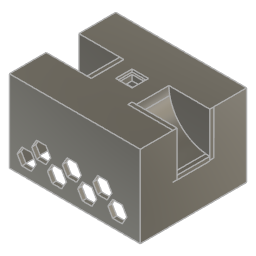
Housing_2_c v4 (Autodesk Fusion 360 archive; units mm, degrees)
design "Housing_2_c"
part number: Configuration 1
Autodesk Fusion 360 part; units mm, degrees
sketch "Sketch1" plane through (0, 0, 0) normal (0, 1, 0) x (1, 0, 0)
  line L0 (0, 0) -> (203.2, 0)
  line L1 (203.2, 0) -> (203.2, -127)
  line L2 (203.2, -127) -> (0, -127)
  line L3 (0, -127) -> (0, 0)
  dimension "d1" = 203.2
  dimension "d2" = 127
  constraint horizontal L0
  constraint vertical L1
  constraint horizontal L2
  constraint vertical L3
  constraint coincident L0.start L3.end
  measures "d1" distance of L0.start L0.end
  measures "d2" distance of L0.start L2.end
extrude "Extrude1" add sketch "Sketch1" along normal blind 165.1
sketch "Sketch3" plane through (0, 0, 0) normal (0, 0, -1) x (1, 0, 0)
  line L0 (203.2, 0) -> (0, 0)
  line L1 (0, 0) -> (0, -165.1)
  line L2 (0, -165.1) -> (203.2, -165.1)
  line L3 (203.2, -165.1) -> (203.2, 0)
  line L4 (6.35, -6.35) -> (196.85, -6.35)
  line L5 (196.85, -6.35) -> (196.85, -158.75)
  line L6 (196.85, -158.75) -> (6.35, -158.75)
  line L7 (6.35, -158.75) -> (6.35, -6.35)
  dimension "d7" = 190.5
  dimension "d8" = 152.4
  dimension "d9" = 6.35
  dimension "d10" = 6.35
  constraint horizontal L4
  constraint vertical L5
  constraint horizontal L6
  constraint vertical L7
  measures "d7" distance of L4.start L4.end
  measures "d8" distance of L4.start L6.end
  measures "d9" distance of L0 L4
  measures "d10" distance of L1 L7
extrude "Extrude2" cut sketch "Sketch3" against normal blind 114.3 contours L4 L5 L6 L7
sketch "Sketch4" plane through (0, 0, 127) normal (0, 0, 1) x (-1, 0, 0)
  line L0 (0, 0) -> (-203.2, 0)
  line L1 (-203.2, 0) -> (-203.2, -165.1)
  line L2 (-203.2, -165.1) -> (0, -165.1)
  line L3 (0, -165.1) -> (0, 0)
  line L4 (-88.9, -101.6) -> (-114.3, -101.6)
  line L5 (-114.3, -101.6) -> (-114.3, -76.2)
  line L6 (-114.3, -76.2) -> (-88.9, -76.2)
  line L7 (-88.9, -76.2) -> (-88.9, -101.6)
  line L8 (-111.125, -79.375) -> (-92.075, -79.375)
  line L9 (-92.075, -79.375) -> (-92.075, -98.425)
  line L10 (-92.075, -98.425) -> (-111.125, -98.425)
  line L11 (-111.125, -98.425) -> (-111.125, -79.375)
  line L12 (-111.125, -79.375) -> (-92.075, -98.425) construction
  line L13 (-92.075, -79.375) -> (-111.125, -98.425) construction
  point P0 (-101.6, -88.9)
  dimension "d13" = 25.4
  dimension "d14" = 25.4
  dimension "d15" = 88.9
  dimension "d16" = 76.2
  dimension "d17" = 19.05
  dimension "d18" = 19.05
  constraint horizontal L4
  constraint vertical L5
  constraint horizontal L6
  constraint vertical L7
  constraint horizontal L8
  constraint perpendicular L8 L9
  constraint parallel L8 L10
  constraint parallel L9 L11
  constraint coincident L12 P0
  constraint coincident L13 P0
  measures "d13" distance of L4.start L4.end
  measures "d14" distance of L4.start L6.end
  measures "d15" distance of L1 L5
  measures "d16" distance of L0 L6
  measures "d17" distance of L9.end L10.end
  measures "d18" distance of L8.end L9.end
extrude "Extrude3" cut sketch "Sketch4" against normal blind 4.064 contours L4 L5 L6 L7
extrude "Extrude4" cut 1 faces at (104.775, 92.075, 127) along direction (0, 0, -1) blind 12.7
ref_plane "WorkPlane1" through (101.6, 82.55, 57.15) normal (0, -1, 0) x (1, 0, 0)
sketch "Sketch5" plane through (0, 82.55, 0) normal (0, -1, 0) x (-1, 0, 0)
  circle A0 centre (-203.2569, -127.0062) radius 63.5
  circle A1 centre (-203.2569, -127.0062) radius 60.325
  dimension "d23" = 127
  dimension "d29" = 120.65
  constraint concentric A0 A1
  measures "d23" diameter of A0
  measures "d29" diameter of A1
extrude "Extrude5" cut sketch "Sketch5" along normal mid plane 50.8 contours A0 | A1
sketch "Sketch6" plane through (0, 82.55, 0) normal (0, -1, 0) x (-1, 0, 0)
  circle A0 centre (0.0225, -126.9197) radius 63.5
  dimension "d26" = 127
  measures "d26" diameter of A0
extrude "Extrude6" cut sketch "Sketch6" along normal mid plane 50.8
sketch "Sketch9" plane through (0, 82.55, 0) normal (0, -1, 0) x (-1, 0, 0)
  arc A0 (-139.7096, -126.9974) -> (-203.216, -63.5038) centre (-203.2096, -127.0038) ccw
  line L0 (-203.2096, -127.0038) -> (-139.7096, -126.9974) construction
  line L1 (-203.2096, -127.0038) -> (-203.216, -63.5038) construction
  line L2 (-203.2096, -127.0038) -> (-146.0596, -126.9981) construction
  line L3 (-203.2096, -127.0038) -> (-203.2154, -69.8538) construction
  arc A1 (-133.3596, -126.9968) -> (-203.2166, -57.1538) centre (-203.2096, -127.0038) ccw
  line L4 (-203.2096, -127.0038) -> (-133.3596, -126.9968) construction
  line L5 (-203.2096, -127.0038) -> (-203.2166, -57.1538) construction
  line L6 (-133.3596, -126.9968) -> (-139.7096, -126.9974)
  line L7 (-203.216, -63.5038) -> (-203.2166, -57.1538)
  dimension "d34" = 63.5
  dimension "d35" = 90
  dimension "d37" = 90
  dimension "d38" = 69.85
  dimension "d39" = 90
  constraint coincident L1 L3.end
  constraint coincident A0.centre L0.start
  constraint parallel L4 L6
  measures "d34" radius of A0
  measures "d35" angle of L0 L1
  measures "d37" angle of L2 L3
  measures "d38" radius of A1
  measures "d39" angle of L4 L5
extrude "Extrude8" add sketch "Sketch9" along normal mid plane 50.8
sketch "Sketch10" plane through (0, 82.55, 0) normal (0, -1, 0) x (-1, 0, 0)
  arc A0 (-0.171, -63.3672) -> (-63.4547, -127.0827) centre (0.0449, -126.8668) ccw
  line L0 (0.0449, -126.8668) -> (-0.171, -63.3672) construction
  line L1 (0.0449, -126.8668) -> (-63.4547, -127.0827) construction
  arc A1 (-0.1926, -57.0172) -> (-69.8047, -127.1043) centre (0.0449, -126.8668) ccw
  line L2 (0.0449, -126.8668) -> (-0.1926, -57.0172) construction
  line L3 (0.0449, -126.8668) -> (-69.8047, -127.1043) construction
  line L4 (-63.4547, -127.0827) -> (-69.8047, -127.1043)
  line L5 (-0.171, -63.3672) -> (-0.1926, -57.0172)
  dimension "d42" = 63.5
  dimension "d43" = 90
  dimension "d44" = 69.85
  dimension "d45" = 90
  constraint coincident A0.centre L0.start
  constraint parallel L3 L4
  measures "d42" radius of A0
  measures "d43" angle of L0 L1
  measures "d44" radius of A1
  measures "d45" angle of L2 L3
extrude "Extrude9" add sketch "Sketch10" along normal mid plane 50.8
sketch "Sketch12" plane through (0, 107.95, 0) normal (0, -1, 0) x (1, 0, 0)
  arc A0 (62.1991, 114.3) -> (63.4549, 127) centre (-0.0449, 126.8668) ccw
  line L0 (63.4549, 127) -> (0, 127)
  line L1 (0, 127) -> (0, 63.4197)
  arc A1 (0, 63.4197) -> (6.35, 63.7403) centre (-0.0225, 126.9197) ccw
  line L2 (6.35, 63.7403) -> (6.35, 114.3)
  line L3 (6.35, 114.3) -> (62.1991, 114.3)
  arc A2 (0.0585, 57.0697) -> (69.8275, 127.0007) centre (-0.0225, 126.9197) ccw
  line L4 (-0.0225, 126.9197) -> (0.0585, 57.0697) construction
  line L5 (-0.0225, 126.9197) -> (69.8275, 127.0007) construction
  line L6 (-0.0225, 126.9197) -> (69.8275, 127.0007)
  line L7 (-0.0225, 126.9197) -> (0.0585, 57.0697)
  dimension "d48" = 69.85
  dimension "d49" = 90
  constraint coincident A1.centre A2.centre
  measures "d48" radius of A2
  measures "d49" angle of L4 L5
sketch "Sketch13" plane through (0, 0, 0) normal (0, -1, 0) x (1, 0, 0)
  line L0 (203.2, 127) -> (0, 127)
  line L1 (0, 127) -> (0, 0)
  line L2 (0, 0) -> (203.2, 0)
  line L3 (203.2, 0) -> (203.2, 127)
  line L4 (34.1009, 12.754) -> (41.4333, 25.454)
  line L5 (41.4333, 25.454) -> (34.1009, 38.154)
  line L6 (34.1009, 38.154) -> (19.4362, 38.154)
  line L7 (19.4362, 38.154) -> (12.1039, 25.454)
  line L8 (12.1039, 25.454) -> (19.4362, 12.754)
  line L9 (19.4362, 12.754) -> (34.1009, 12.754)
  point P0 (26.7686, 25.454)
  dimension "d55" = 12.7
  constraint parallel L2 L9
  measures "d55" distance of P0 L9
extrude "Extrude12" cut sketch "Sketch13" against normal blind 6.35 contours L4 L5 L6 L7 L8 L9
pattern_linear "R-Pattern1" count 4 spacing 46.99 along (1, 0, 0) of "Extrude12"
sketch "Sketch14" plane through (0, 0, 0) normal (0, -1, 0) x (1, 0, 0)
  line L0 (182.4033, 25.454) -> (175.0709, 12.754)
  line L1 (175.0709, 12.754) -> (160.4062, 12.754)
  line L2 (160.4062, 12.754) -> (153.0739, 25.454)
  line L3 (153.0739, 25.454) -> (160.4062, 38.154)
  line L4 (160.4062, 38.154) -> (175.0709, 38.154)
  line L5 (175.0709, 38.154) -> (182.4033, 25.454)
  line L6 (135.4133, 25.454) -> (128.0809, 12.754)
  line L7 (128.0809, 12.754) -> (113.4162, 12.754)
  line L8 (113.4162, 12.754) -> (106.0839, 25.454)
  line L9 (106.0839, 25.454) -> (113.4162, 38.154)
  line L10 (113.4162, 38.154) -> (128.0809, 38.154)
  line L11 (128.0809, 38.154) -> (135.4133, 25.454)
  line L12 (88.4233, 25.454) -> (81.0909, 12.754)
  line L13 (81.0909, 12.754) -> (66.4262, 12.754)
  line L14 (66.4262, 12.754) -> (59.0939, 25.454)
  line L15 (59.0939, 25.454) -> (66.4262, 38.154)
  line L16 (66.4262, 38.154) -> (81.0909, 38.154)
  line L17 (81.0909, 38.154) -> (88.4233, 25.454)
  line L18 (41.4333, 25.454) -> (34.1009, 12.754)
  line L19 (34.1009, 12.754) -> (19.4362, 12.754)
  line L20 (19.4362, 12.754) -> (12.1039, 25.454)
  line L21 (12.1039, 25.454) -> (19.4362, 38.154)
  line L22 (19.4362, 38.154) -> (34.1009, 38.154)
  line L23 (34.1009, 38.154) -> (41.4333, 25.454)
  line L24 (203.2, 127) -> (0, 127)
  line L25 (0, 127) -> (0, 0)
  line L26 (0, 0) -> (203.2, 0)
  line L27 (203.2, 0) -> (203.2, 127)
  line L28 (56.7841, 58.6176) -> (42.1194, 58.6216)
  line L29 (42.1194, 58.6216) -> (34.7835, 45.9236)
  line L30 (34.7835, 45.9236) -> (42.1124, 33.2216)
  line L31 (42.1124, 33.2216) -> (56.7771, 33.2176)
  line L32 (56.7771, 33.2176) -> (64.1129, 45.9155)
  line L33 (64.1129, 45.9155) -> (56.7841, 58.6176)
  point P0 (49.4482, 45.9196)
  dimension "d62" = 12.7
  measures "d62" distance of P0 L33
extrude "Extrude13" cut sketch "Sketch14" against normal blind 6.35 contours L28 L29 L30 L31 L32 L33
pattern_linear "R-Pattern2" count 3 spacing 47.4726 along (1, 0, 0) of "Extrude13"
sketch "Sketch15" plane through (0, 165.1, 0) normal (0, 1, 0) x (-1, 0, 0)
  line L0 (0, 127) -> (-203.2, 127)
  line L1 (-203.2, 127) -> (-203.2, 0)
  line L2 (-203.2, 0) -> (0, 0)
  line L3 (0, 0) -> (0, 127)
  line L4 (-35.8949, 19.9662) -> (-21.2302, 19.954)
  line L5 (-21.2302, 19.954) -> (-13.8872, 32.6478)
  line L6 (-13.8872, 32.6478) -> (-21.2089, 45.3539)
  line L7 (-21.2089, 45.3539) -> (-35.8736, 45.3662)
  line L8 (-35.8736, 45.3662) -> (-43.2166, 32.6724)
  line L9 (-43.2166, 32.6724) -> (-35.8949, 19.9662)
  point P0 (-28.5519, 32.6601)
  dimension "d69" = 12.7
  measures "d69" distance of P0 L9
extrude "Extrude14" cut sketch "Sketch15" against normal blind 6.35 contours L4 L5 L6 L7 L8 L9
pattern_linear "R-Pattern3" count 4 spacing 47.9467 along (1, 0, 0) of "Extrude14"
sketch "Sketch16" plane through (0, 165.1, 0) normal (0, 1, 0) x (-1, 0, 0)
  line L0 (-165.0704, 19.954) -> (-179.7351, 19.9662)
  line L1 (-179.7351, 19.9662) -> (-187.0568, 32.6724)
  line L2 (-187.0568, 32.6724) -> (-179.7138, 45.3662)
  line L3 (-179.7138, 45.3662) -> (-165.0491, 45.3539)
  line L4 (-165.0491, 45.3539) -> (-157.7274, 32.6478)
  line L5 (-157.7274, 32.6478) -> (-165.0704, 19.954)
  line L6 (-117.1237, 19.954) -> (-131.7884, 19.9662)
  line L7 (-131.7884, 19.9662) -> (-139.1101, 32.6724)
  line L8 (-139.1101, 32.6724) -> (-131.7671, 45.3662)
  line L9 (-131.7671, 45.3662) -> (-117.1024, 45.3539)
  line L10 (-117.1024, 45.3539) -> (-109.7807, 32.6478)
  line L11 (-109.7807, 32.6478) -> (-117.1237, 19.954)
  line L12 (-69.1769, 19.954) -> (-83.8416, 19.9662)
  line L13 (-83.8416, 19.9662) -> (-91.1633, 32.6724)
  line L14 (-91.1633, 32.6724) -> (-83.8203, 45.3662)
  line L15 (-83.8203, 45.3662) -> (-69.1557, 45.3539)
  line L16 (-69.1557, 45.3539) -> (-61.834, 32.6478)
  line L17 (-61.834, 32.6478) -> (-69.1769, 19.954)
  line L18 (-21.2302, 19.954) -> (-35.8949, 19.9662)
  line L19 (-35.8949, 19.9662) -> (-43.2166, 32.6724)
  line L20 (-43.2166, 32.6724) -> (-35.8736, 45.3662)
  line L21 (-35.8736, 45.3662) -> (-21.2089, 45.3539)
  line L22 (-21.2089, 45.3539) -> (-13.8872, 32.6478)
  line L23 (-13.8872, 32.6478) -> (-21.2302, 19.954)
  line L24 (0, 127) -> (-203.2, 127)
  line L25 (-203.2, 127) -> (-203.2, 0)
  line L26 (-203.2, 0) -> (0, 0)
  line L27 (0, 0) -> (0, 127)
  line L28 (-59.9209, 36.6353) -> (-45.2566, 36.5385)
  line L29 (-45.2566, 36.5385) -> (-37.8405, 49.1898)
  line L30 (-37.8405, 49.1898) -> (-45.0888, 61.9379)
  line L31 (-45.0888, 61.9379) -> (-59.7532, 62.0348)
  line L32 (-59.7532, 62.0348) -> (-67.1692, 49.3835)
  line L33 (-67.1692, 49.3835) -> (-59.9209, 36.6353)
  point P0 (-52.5049, 49.2866)
  dimension "d76" = 12.7
  measures "d76" distance of P0 L33
extrude "Extrude15" cut sketch "Sketch16" against normal blind 6.35 contours L28 L29 L30 L31 L32 L33
pattern_linear "R-Pattern4" count 3 spacing 47.9806 along (1, 0, 0) of "Extrude15"
extrude "Extrude16" add sketch "Sketch12" against normal blind 6.35 contours A0 L1 A1 L2 L3 L6 L7 | A0 A1 L2 L3 A2 L6 L7
ref_plane "WorkPlane3" through (31.7342, 57.15, 95.2098) normal (0, 1, 0) x (1, 0, 0)
sketch "Sketch20" plane through (0, 57.15, 0) normal (0, 1, 0) x (1, 0, 0)
  arc A0 (69.8539, -126.9924) -> (0.2121, -56.9348) centre (0.0042, -126.7845) ccw
  line L0 (0.0042, -126.7845) -> (69.8539, -126.9924) construction
  line L1 (0.0042, -126.7845) -> (0.2121, -56.9348) construction
  line L2 (69.8539, -126.9924) -> (0.0042, -126.7845)
  line L3 (0.0042, -126.7845) -> (0.2121, -56.9348)
  dimension "d91" = 69.85
  dimension "d92" = 90
  constraint coincident A0.centre L0.start
  measures "d91" radius of A0
  measures "d92" angle of L0 L1
extrude "Extrude18" add sketch "Sketch20" against normal blind 6.35
ref_plane "WorkPlane4" through (171.4785, 107.95, 95.2531) normal (0, -1, 0) x (-1, 0, 0)
sketch "Sketch22" plane through (0, 107.95, 0) normal (0, -1, 0) x (-1, 0, 0)
  arc A0 (-133.4095, -126.9653) -> (-203.1991, -57.055) centre (-203.2595, -126.905) ccw
  line L0 (-203.2595, -126.905) -> (-133.4095, -126.9653) construction
  line L1 (-203.2595, -126.905) -> (-203.1991, -57.055) construction
  line L2 (-133.4095, -126.9653) -> (-203.2595, -126.905)
  line L3 (-203.2595, -126.905) -> (-203.1991, -57.055)
  dimension "d96" = 69.85
  dimension "d97" = 90
  constraint coincident A0.centre L0.start
  measures "d96" radius of A0
  measures "d97" angle of L0 L1
extrude "Extrude19" add sketch "Sketch22" against normal blind 6.35
ref_plane "WorkPlane5" through (171.4785, 57.15, 95.2531) normal (0, 1, 0) x (1, 0, 0)
sketch "Sketch23" plane through (0, 57.15, 0) normal (0, 1, 0) x (1, 0, 0)
  arc A0 (203.0491, -57.1406) -> (133.3432, -127.1344) centre (203.1931, -126.9905) ccw
  line L0 (203.1931, -126.9905) -> (203.0491, -57.1406) construction
  line L1 (203.1931, -126.9905) -> (133.3432, -127.1344) construction
  line L2 (133.3432, -127.1344) -> (203.1931, -126.9905)
  line L3 (203.1931, -126.9905) -> (203.0491, -57.1406)
  dimension "d101" = 69.85
  dimension "d102" = 90
  constraint coincident A0.centre L0.start
  measures "d101" radius of A0
  measures "d102" angle of L0 L1
extrude "Extrude20" cut sketch "Sketch23" against normal blind 6.35
ref_plane "WorkPlane6" through (168.2676, 50.8, 92.0703) normal (0, 1, 0) x (1, 0, 0)
sketch "Sketch24" plane through (0, 50.8, 0) normal (0, 1, 0) x (1, 0, 0)
  arc A0 (203.1979, -57.15) -> (133.3479, -127) centre (203.1979, -127) ccw
  line L0 (203.1979, -127) -> (203.1979, -57.15) construction
  line L1 (203.1979, -127) -> (133.3479, -127) construction
  line L2 (133.3479, -127) -> (203.1979, -127)
  line L3 (203.1979, -127) -> (203.1979, -57.15)
  dimension "d106" = 69.85
  dimension "d107" = 90
  constraint coincident A0.centre L0.start
  measures "d106" radius of A0
  measures "d107" angle of L0 L1
extrude "Extrude21" add sketch "Sketch24" along normal blind 6.35
delete_face "DeleteFace2" 4 faces at (69.82, 107.95, 127.0001) (69.8275, 112.1833, 127.0006) (69.6354, 114.3, 127.0004) (69.6278, 112.1833, 127.0004)
